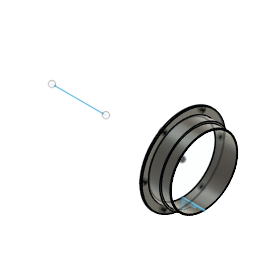
outlet duct adapter (Autodesk Fusion 360 design; units mm, degrees)
Autodesk Fusion 360 part; units mm, degrees
sketch "sketch 650" plane through (0, -71.146, 0) normal (0, 1, 0) x (1, 0, 0)
  line L0 (194.6, 32.5398) -> (198.6, 32.5398)
  line L1 (194.6, 32.5398) -> (173.6, 32.5398)
  line L2 (173.6, 47.5398) -> (173.6, 32.5398)
  line L3 (169.6, 47.5398) -> (173.6, 47.5398)
  line L4 (169.6, 27.9253) -> (169.6, 47.5398)
  line L5 (169.6, 27.9253) -> (170.4854, 27.0398)
  line L6 (170.4854, 27.0398) -> (218.6, 27.0398)
  line L7 (218.6, 29.0398) -> (218.6, 27.0398)
  line L8 (198.6, 29.0398) -> (218.6, 29.0398)
  line L9 (198.6, 32.5398) -> (198.6, 29.0398)
revolve "Revolve1" add sketch "sketch 650" angle 360 about axis through (0, -71.146, 46.1602) along (-1, 0, 0)
sketch "Sketch1" plane through (169.6, 0, 0) normal (-1, 0, 0) x (0, -1, 0)
  circle A0 centre (71.146, 46.1602) radius 74.0854
  circle A1 centre (71.146, 46.1602) radius 93.7
  circle A2 centre (114.146, -28.318) radius 1.6
  circle A3 centre (157.146, 46.1602) radius 1.6
  circle A4 centre (114.146, 120.6384) radius 1.6
  circle A5 centre (28.146, 120.6384) radius 1.6
  circle A6 centre (-14.854, 46.1602) radius 1.6
  circle A7 centre (28.146, -28.318) radius 1.6
  point P0 (71.146, 46.1602)
  dimension "d195" = 360
extrude "Extrude1" cut sketch "Sketch1" against normal up to surface (4 mm away) contours A2 | A3 | A4 | A5 | A6 | A7
chamfer "Chamfer1" distance 0.6 angle 45 9 edges at (173.6, -105.0293, 133.5193) (169.6, -105.0293, 133.5193) (169.6, -26.6543, -27.7394) (169.6, 16.3457, 46.7388) (169.6, -26.6543, 121.217) (169.6, -112.6543, 121.217) (169.6, -155.6543, 46.7388) (169.6, -112.6543, -27.7394) (218.6, -98.3395, 116.2712)
named bodies: "outlet duct"
